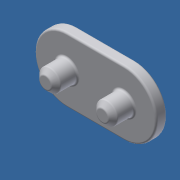
# Autodesk Inventor part: J005537
Saved by Autodesk Inventor 2018.2 (Build 222227000, 227)
## iProperties
Created: 2014-10-13
Material: VERO WHITE
Vendor: HHMI: JFRC - ID&F
Document SubType Name: Modeling
Designer: negrashovi
Density: 1.17 g/cm^3
Project: P-75301
Part Number: J005537
Description: SUPPORT FOR ROUND INSERT
Mass: 0.0352257 g
Surface Area: 0.919099 cm^2
Volume: 0.0301074 cm^3
Appearance: Plastic (White)
RuleStatus: InUse
AfterDocSave0: file://Part Number Cleaner
LAB/DEPT: RUBIN (LAB)
REQUESTING SCIENTIST: ASO, YOSHI
SURFACE ROUGHNESS: N/A
DESIGN DEPARTMENT: HHMI: JRC - ID&F
SPECIAL FINISH: NONE
ALTERED ITEM PART NUMBER: N/A
ALTERED ITEM VENDOR: N/A
ALTERED ITEM DESCRIPTION: N/A
Author: negrashovi
Revision Number: A
Autodesk Inventor part; units mm, degrees
ref_plane "YZ Plane" through (0, 0, 0) normal (1, 0, 0) x (0, 1, 0)
ref_plane "XZ Plane" through (0, 0, 0) normal (0, 1, 0) x (-1, 0, 0)
ref_plane "XY Plane" through (0, 0, 0) normal (0, 0, 1) x (1, 0, 0)
sketch "Sketch1" plane through (0, 0, 0) normal (0, 0, 1) x (1, 0, 0)
  arc A0 (-1.846, 54.9588) -> (-1.846, 50.7678) centre (-1.846, 52.8633) ccw
  arc A1 (1.846, 50.7678) -> (1.846, 54.9588) centre (1.846, 52.8633) ccw
  line L0 (0, -74.4664) -> (0, 76.5296) construction
  line L1 (-74.0537, 0) -> (74.0537, 0) construction
  circle A2 centre (0, 0) radius 52.8955 construction
  circle A3 centre (-1.846, 52.8633) radius 0.7
  circle A4 centre (1.846, 52.8633) radius 0.7
  line L2 (-1.846, 54.9588) -> (1.846, 54.9588)
  line L3 (-1.846, 50.7678) -> (1.846, 50.7678)
  dimension "d3" = 1.4
  dimension "d4" = 4
  dimension "d12" = 4.191
  dimension "d13" = 105.791
  constraints: 7 point on circle, 5 centre point, 4 end point, 2 coincident, 2 tangent, 1 parallel, 1 perpendicular, 2 other
  measures "d3" diameter of A4
  measures "d12" distance between parallel lines of L3 L2
  measures "d13" diameter of A2
extrude "Extrusion1" add sketch "Sketch1" against normal blind 0.7 contours L2 A1 L3 A0 | A3 | A4
extrude "Extrusion2" add sketch "Sketch1" along normal blind 1.4 contours A3 | A4
chamfer "Chamfer1" distance 0.3048 angle 45 2 edges at (-2.546, 52.8633, 1.4) (1.146, 52.8633, 1.4)
fillet "Fillet1" radius 0.127 14 edges at (0, 54.9588, 0) (3.9415, 52.8633, 0) (0, 50.7678, 0) (-3.9415, 52.8633, 0) (0, 50.7678, -0.7) (3.9415, 52.8633, -0.7) (0, 54.9588, -0.7) (-3.9415, 52.8633, -0.7) (-2.546, 52.8633, 0) (1.146, 52.8633, 0) (1.146, 52.8633, 1.0952) (1.4508, 52.8633, 1.4) (-2.546, 52.8633, 1.0952) (-2.2412, 52.8633, 1.4)
body "Solid1"
